Autodesk Fusion 360 part; units mm, degrees
note: some values were not read from the file. Chosen so that the rebuilt part matches the saved one: a direction. Set by a fixed rule: which sketch regions a step uses.
(part 2 of 8)
  arc A22 (27.5172, -41.7722) -> (27.7255, -40.9948) centre (13.5, -37.5997) ccw
  spline S11 degree 5 poles (27.7255, -40.9948) (27.7209, -40.9905) (27.7118, -40.9819) (27.698, -40.969) (27.6796, -40.952) (27.6566, -40.9308) (27.6336, -40.9097) (27.6104, -40.8888) (27.5872, -40.868) (27.564, -40.8473) (27.5406, -40.8268) (27.5173, -40.8064) (27.4938, -40.7861) (27.4703, -40.766) (27.4468, -40.746) (27.4232, -40.7262) (27.3995, -40.7065) (27.3758, -40.6869) (27.352, -40.6675) (27.3281, -40.6482) (27.3042, -40.6291) (27.2803, -40.6101) (27.2562, -40.5912) (27.2321, -40.5725) (27.208, -40.554) (27.1838, -40.5356) (27.1595, -40.5174) (27.1352, -40.4993) (27.1108, -40.4813) (27.0864, -40.4636) (27.0619, -40.4459) (27.0374, -40.4285) (27.0128, -40.4112) (26.9881, -40.394) (26.9634, -40.377) (26.9386, -40.3602) (26.9138, -40.3436) (26.8889, -40.3271) (26.8639, -40.3108) (26.8389, -40.2947) (26.8138, -40.2787) (26.7887, -40.2629) (26.7635, -40.2474) (26.7382, -40.232) (26.7129, -40.2167) (26.6876, -40.2017) (26.6621, -40.1869) (26.6367, -40.1722) (26.6111, -40.1577) (26.5855, -40.1435) (26.5599, -40.1294) (26.5341, -40.1156) (26.5083, -40.102) (26.4825, -40.0886) (26.4566, -40.0755) (26.4306, -40.0626) (26.4046, -40.0498) (26.3785, -40.0373) (26.3523, -40.025) (26.3261, -40.013) (26.2998, -40.0012) (26.2734, -39.9898) (26.247, -39.9788) (26.2204, -39.9682) (26.1937, -39.9578) (26.167, -39.9477) (26.1403, -39.9378) (26.1135, -39.9281) (26.0867, -39.9186) (26.0598, -39.9097) (26.0327, -39.9015) (26.0108, -39.8958) (25.9943, -39.8921) (25.9832, -39.8899) (25.9776, -39.8889) knots -1 -1 -1 -1 -1 -1 -0.98571429 -0.97142857 -0.95714286 -0.94285714 -0.92857143 -0.91428571 -0.9 -0.88571429 -0.87142857 -0.85714286 -0.84285714 -0.82857143 -0.81428571 -0.8 -0.78571429 -0.77142857 -0.75714286 -0.74285714 -0.72857143 -0.71428571 -0.7 -0.68571429 -0.67142857 -0.65714286 -0.64285714 -0.62857143 -0.61428571 -0.6 -0.58571429 -0.57142857 -0.55714286 -0.54285714 -0.52857143 -0.51428571 -0.5 -0.48571429 -0.47142857 -0.45714286 -0.44285714 -0.42857143 -0.41428571 -0.4 -0.38571429 -0.37142857 -0.35714286 -0.34285714 -0.32857143 -0.31428571 -0.3 -0.28571429 -0.27142857 -0.25714286 -0.24285714 -0.22857143 -0.21428571 -0.2 -0.18571429 -0.17142857 -0.15714286 -0.14285714 -0.12857143 -0.11428571 -0.1 -0.08571429 -0.07142857 -0.05714286 -0.04285714 -0.02857143 -0.01428571 0 0 0 0 0 0
  line L11 (25.9776, -39.8889) -> (25.5961, -39.8189)
  arc A23 (25.5156, -39.7033) -> (25.5961, -39.8189) centre (25.6141, -39.7205) ccw
  arc A24 (25.5156, -39.7033) -> (25.6507, -38.6777) centre (13.5, -37.5997) ccw
  arc A25 (25.7583, -38.5868) -> (25.6507, -38.6777) centre (25.7503, -38.6865) ccw
  line L12 (25.7583, -38.5868) -> (26.1449, -38.618)
  spline S12 degree 5 poles (26.1449, -38.618) (26.1506, -38.6184) (26.1618, -38.6192) (26.1788, -38.6199) (26.2014, -38.6201) (26.2297, -38.6192) (26.258, -38.6175) (26.2864, -38.6153) (26.3147, -38.6128) (26.3431, -38.6102) (26.3715, -38.6073) (26.3999, -38.6043) (26.4284, -38.6008) (26.4568, -38.5971) (26.4852, -38.5929) (26.5137, -38.5883) (26.5421, -38.5835) (26.5705, -38.5784) (26.599, -38.573) (26.6274, -38.5675) (26.6559, -38.5617) (26.6843, -38.5557) (26.7127, -38.5495) (26.7412, -38.5431) (26.7696, -38.5364) (26.798, -38.5294) (26.8264, -38.5223) (26.8549, -38.5149) (26.8833, -38.5073) (26.9117, -38.4996) (26.9401, -38.4916) (26.9684, -38.4835) (26.9968, -38.4751) (27.0252, -38.4666) (27.0535, -38.4579) (27.0819, -38.4489) (27.1102, -38.4398) (27.1385, -38.4305) (27.1669, -38.4211) (27.1952, -38.4114) (27.2234, -38.4016) (27.2517, -38.3916) (27.28, -38.3814) (27.3082, -38.3711) (27.3365, -38.3606) (27.3647, -38.3499) (27.3929, -38.339) (27.4211, -38.328) (27.4492, -38.3168) (27.4774, -38.3055) (27.5055, -38.294) (27.5337, -38.2823) (27.5618, -38.2705) (27.5898, -38.2585) (27.6179, -38.2464) (27.646, -38.2341) (27.674, -38.2216) (27.702, -38.209) (27.73, -38.1963) (27.7579, -38.1834) (27.7859, -38.1703) (27.8138, -38.1571) (27.8417, -38.1437) (27.8696, -38.1302) (27.8975, -38.1166) (27.9253, -38.1028) (27.9531, -38.0889) (27.9809, -38.0748) (28.0087, -38.0605) (28.0364, -38.0462) (28.0641, -38.0317) (28.0863, -38.0199) (28.1029, -38.0111) (28.1139, -38.0051) (28.1195, -38.0022) knots 0 0 0 0 0 0 0.01428571 0.02857143 0.04285714 0.05714286 0.07142857 0.08571429 0.1 0.11428571 0.12857143 0.14285714 0.15714286 0.17142857 0.18571429 0.2 0.21428571 0.22857143 0.24285714 0.25714286 0.27142857 0.28571429 0.3 0.31428571 0.32857143 0.34285714 0.35714286 0.37142857 0.38571429 0.4 0.41428571 0.42857143 0.44285714 0.45714286 0.47142857 0.48571429 0.5 0.51428571 0.52857143 0.54285714 0.55714286 0.57142857 0.58571429 0.6 0.61428571 0.62857143 0.64285714 0.65714286 0.67142857 0.68571429 0.7 0.71428571 0.72857143 0.74285714 0.75714286 0.77142857 0.78571429 0.8 0.81428571 0.82857143 0.84285714 0.85714286 0.87142857 0.88571429 0.9 0.91428571 0.92857143 0.94285714 0.95714286 0.97142857 0.98571429 1 1 1 1 1 1
  arc A26 (28.1195, -38.0022) -> (28.1195, -37.1973) centre (13.5, -37.5997) ccw
  spline S13 degree 5 poles (28.1195, -37.1973) (28.1139, -37.1943) (28.1029, -37.1884) (28.0863, -37.1795) (28.0641, -37.1678) (28.0364, -37.1533) (28.0087, -37.1389) (27.9809, -37.1247) (27.9531, -37.1106) (27.9253, -37.0966) (27.8975, -37.0828) (27.8696, -37.0692) (27.8417, -37.0557) (27.8138, -37.0423) (27.7859, -37.0291) (27.7579, -37.0161) (27.73, -37.0032) (27.702, -36.9904) (27.674, -36.9778) (27.646, -36.9653) (27.6179, -36.9531) (27.5898, -36.9409) (27.5618, -36.9289) (27.5337, -36.9171) (27.5055, -36.9054) (27.4774, -36.8939) (27.4492, -36.8826) (27.4211, -36.8714) (27.3929, -36.8604) (27.3647, -36.8495) (27.3365, -36.8389) (27.3082, -36.8283) (27.28, -36.818) (27.2517, -36.8078) (27.2234, -36.7978) (27.1952, -36.788) (27.1669, -36.7784) (27.1385, -36.7689) (27.1102, -36.7596) (27.0819, -36.7505) (27.0535, -36.7416) (27.0252, -36.7328) (26.9968, -36.7243) (26.9684, -36.716) (26.9401, -36.7078) (26.9117, -36.6999) (26.8833, -36.6921) (26.8549, -36.6845) (26.8264, -36.6772) (26.798, -36.67) (26.7696, -36.6631) (26.7412, -36.6564) (26.7127, -36.6499) (26.6843, -36.6437) (26.6559, -36.6377) (26.6274, -36.632) (26.599, -36.6264) (26.5705, -36.6211) (26.5421, -36.6159) (26.5137, -36.6111) (26.4852, -36.6066) (26.4568, -36.6024) (26.4284, -36.5986) (26.3999, -36.5952) (26.3715, -36.5921) (26.3431, -36.5893) (26.3147, -36.5866) (26.2864, -36.5841) (26.258, -36.5819) (26.2297, -36.5802) (26.2014, -36.5793) (26.1788, -36.5795) (26.1618, -36.5802) (26.1506, -36.581) (26.1449, -36.5815) knots -1 -1 -1 -1 -1 -1 -0.98571429 -0.97142857 -0.95714286 -0.94285714 -0.92857143 -0.91428571 -0.9 -0.88571429 -0.87142857 -0.85714286 -0.84285714 -0.82857143 -0.81428571 -0.8 -0.78571429 -0.77142857 -0.75714286 -0.74285714 -0.72857143 -0.71428571 -0.7 -0.68571429 -0.67142857 -0.65714286 -0.64285714 -0.62857143 -0.61428571 -0.6 -0.58571429 -0.57142857 -0.55714286 -0.54285714 -0.52857143 -0.51428571 -0.5 -0.48571429 -0.47142857 -0.45714286 -0.44285714 -0.42857143 -0.41428571 -0.4 -0.38571429 -0.37142857 -0.35714286 -0.34285714 -0.32857143 -0.31428571 -0.3 -0.28571429 -0.27142857 -0.25714286 -0.24285714 -0.22857143 -0.21428571 -0.2 -0.18571429 -0.17142857 -0.15714286 -0.14285714 -0.12857143 -0.11428571 -0.1 -0.08571429 -0.07142857 -0.05714286 -0.04285714 -0.02857143 -0.01428571 0 0 0 0 0 0
  line L13 (26.1449, -36.5815) -> (25.7583, -36.6126)
  arc A27 (25.6507, -36.5217) -> (25.7583, -36.6126) centre (25.7503, -36.5129) ccw
  arc A28 (25.6507, -36.5217) -> (25.5156, -35.4961) centre (13.5, -37.5997) ccw
  arc A29 (25.5961, -35.3805) -> (25.5156, -35.4961) centre (25.6141, -35.4789) ccw
  line L14 (25.5961, -35.3805) -> (25.9776, -35.3105)
  spline S14 degree 5 poles (25.9776, -35.3105) (25.9832, -35.3095) (25.9943, -35.3073) (26.0108, -35.3037) (26.0327, -35.298) (26.0598, -35.2898) (26.0867, -35.2808) (26.1135, -35.2713) (26.1403, -35.2616) (26.167, -35.2517) (26.1937, -35.2416) (26.2204, -35.2313) (26.247, -35.2206) (26.2734, -35.2096) (26.2998, -35.1982) (26.3261, -35.1865) (26.3523, -35.1744) (26.3785, -35.1621) (26.4046, -35.1496) (26.4306, -35.1369) (26.4566, -35.124) (26.4825, -35.1108) (26.5083, -35.0974) (26.5341, -35.0838) (26.5599, -35.07) (26.5855, -35.056) (26.6111, -35.0417) (26.6367, -35.0272) (26.6621, -35.0126) (26.6876, -34.9977) (26.7129, -34.9827) (26.7382, -34.9675) (26.7635, -34.9521) (26.7887, -34.9365) (26.8138, -34.9207) (26.8389, -34.9048) (26.8639, -34.8886) (26.8889, -34.8723) (26.9138, -34.8558) (26.9386, -34.8392) (26.9634, -34.8224) (26.9881, -34.8054) (27.0128, -34.7883) (27.0374, -34.771) (27.0619, -34.7535) (27.0864, -34.7359) (27.1108, -34.7181) (27.1352, -34.7002) (27.1595, -34.6821) (27.1838, -34.6638) (27.208, -34.6454) (27.2321, -34.6269) (27.2562, -34.6082) (27.2803, -34.5894) (27.3042, -34.5704) (27.3281, -34.5512) (27.352, -34.5319) (27.3758, -34.5125) (27.3995, -34.493) (27.4232, -34.4733) (27.4468, -34.4534) (27.4703, -34.4334) (27.4938, -34.4133) (27.5173, -34.393) (27.5406, -34.3726) (27.564, -34.3521) (27.5872, -34.3315) (27.6104, -34.3107) (27.6336, -34.2897) (27.6566, -34.2687) (27.6796, -34.2475) (27.698, -34.2304) (27.7118, -34.2176) (27.7209, -34.209) (27.7255, -34.2047) knots 0 0 0 0 0 0 0.01428571 0.02857143 0.04285714 0.05714286 0.07142857 0.08571429 0.1 0.11428571 0.12857143 0.14285714 0.15714286 0.17142857 0.18571429 0.2 0.21428571 0.22857143 0.24285714 0.25714286 0.27142857 0.28571429 0.3 0.31428571 0.32857143 0.34285714 0.35714286 0.37142857 0.38571429 0.4 0.41428571 0.42857143 0.44285714 0.45714286 0.47142857 0.48571429 0.5 0.51428571 0.52857143 0.54285714 0.55714286 0.57142857 0.58571429 0.6 0.61428571 0.62857143 0.64285714 0.65714286 0.67142857 0.68571429 0.7 0.71428571 0.72857143 0.74285714 0.75714286 0.77142857 0.78571429 0.8 0.81428571 0.82857143 0.84285714 0.85714286 0.87142857 0.88571429 0.9 0.91428571 0.92857143 0.94285714 0.95714286 0.97142857 0.98571429 1 1 1 1 1 1
  arc A30 (27.7255, -34.2047) -> (27.5172, -33.4272) centre (13.5, -37.5997) ccw
  spline S15 degree 5 poles (27.5172, -33.4272) (27.511, -33.4257) (27.4988, -33.4229) (27.4805, -33.4186) (27.4561, -33.413) (27.4255, -33.4062) (27.395, -33.3995) (27.3645, -33.3929) (27.334, -33.3865) (27.3036, -33.3802) (27.2731, -33.3741) (27.2427, -33.3681) (27.2122, -33.3623) (27.1818, -33.3566) (27.1514, -33.3511) (27.1211, -33.3457) (27.0907, -33.3405) (27.0604, -33.3354) (27.03, -33.3305) (26.9998, -33.3257) (26.9695, -33.3211) (26.9392, -33.3166) (26.909, -33.3123) (26.8788, -33.3082) (26.8486, -33.3042) (26.8185, -33.3004) (26.7883, -33.2967) (26.7582, -33.2932) (26.7281, -33.2898) (26.6981, -33.2867) (26.6681, -33.2836) (26.6381, -33.2808) (26.6081, -33.2781) (26.5782, -33.2756) (26.5483, -33.2733) (26.5184, -33.2711) (26.4886, -33.2691) (26.4588, -33.2673) (26.429, -33.2656) (26.3993, -33.2642) (26.3696, -33.2629) (26.34, -33.2618) (26.3103, -33.2609) (26.2808, -33.2602) (26.2512, -33.2597) (26.2218, -33.2593) (26.1923, -33.2592) (26.1629, -33.2592) (26.1336, -33.2595) (26.1043, -33.2599) (26.075, -33.2606) (26.0458, -33.2615) (26.0167, -33.2626) (25.9876, -33.2639) (25.9586, -33.2655) (25.9296, -33.2673) (25.9007, -33.2693) (25.8719, -33.2715) (25.8431, -33.2739) (25.8144, -33.2766) (25.7857, -33.2796) (25.7572, -33.2829) (25.7287, -33.2866) (25.7004, -33.2907) (25.6722, -33.295) (25.644, -33.2996) (25.6159, -33.3044) (25.5878, -33.3094) (25.5599, -33.3146) (25.5321, -33.3203) (25.5045, -33.3267) (25.4827, -33.3328) (25.4665, -33.3378) (25.4558, -33.3415) (25.4505, -33.3434) knots -1 -1 -1 -1 -1 -1 -0.98571429 -0.97142857 -0.95714286 -0.94285714 -0.92857143 -0.91428571 -0.9 -0.88571429 -0.87142857 -0.85714286 -0.84285714 -0.82857143 -0.81428571 -0.8 -0.78571429 -0.77142857 -0.75714286 -0.74285714 -0.72857143 -0.71428571 -0.7 -0.68571429 -0.67142857 -0.65714286 -0.64285714 -0.62857143 -0.61428571 -0.6 -0.58571429 -0.57142857 -0.55714286 -0.54285714 -0.52857143 -0.51428571 -0.5 -0.48571429 -0.47142857 -0.45714286 -0.44285714 -0.42857143 -0.41428571 -0.4 -0.38571429 -0.37142857 -0.35714286 -0.34285714 -0.32857143 -0.31428571 -0.3 -0.28571429 -0.27142857 -0.25714286 -0.24285714 -0.22857143 -0.21428571 -0.2 -0.18571429 -0.17142857 -0.15714286 -0.14285714 -0.12857143 -0.11428571 -0.1 -0.08571429 -0.07142857 -0.05714286 -0.04285714 -0.02857143 -0.01428571 0 0 0 0 0 0
  line L15 (25.4505, -33.3434) -> (25.0851, -33.4735)
  arc A31 (24.9576, -33.4137) -> (25.0851, -33.4735) centre (25.0516, -33.3793) ccw
  arc A32 (24.9576, -33.4137) -> (24.5618, -32.4579) centre (13.5, -37.5997) ccw
  arc A33 (24.6096, -32.3255) -> (24.5618, -32.4579) centre (24.6524, -32.4158) ccw
  line L16 (24.6096, -32.3255) -> (24.96, -32.1591)
  spline S16 degree 5 poles (24.96, -32.1591) (24.9651, -32.1567) (24.9752, -32.1517) (24.9903, -32.1439) (25.0099, -32.1327) (25.034, -32.1178) (25.0577, -32.1021) (25.0811, -32.086) (25.1045, -32.0697) (25.1277, -32.0532) (25.1509, -32.0366) (25.174, -32.0197) (25.1969, -32.0025) (25.2196, -31.985) (25.2421, -31.9672) (25.2645, -31.9491) (25.2867, -31.9306) (25.3087, -31.912) (25.3307, -31.8931) (25.3526, -31.8741) (25.3743, -31.8549) (25.3959, -31.8355) (25.4175, -31.8159) (25.4389, -31.7961) (25.4601, -31.7761) (25.4813, -31.7559) (25.5023, -31.7355) (25.5232, -31.7149) (25.5441, -31.6941) (25.5648, -31.6732) (25.5854, -31.6521) (25.6059, -31.6309) (25.6263, -31.6094) (25.6466, -31.5879) (25.6668, -31.5661) (25.6869, -31.5442) (25.7069, -31.5222) (25.7267, -31.5) (25.7465, -31.4776) (25.7662, -31.4551) (25.7858, -31.4324) (25.8053, -31.4096) (25.8247, -31.3867) (25.844, -31.3636) (25.8632, -31.3404) (25.8822, -31.317) (25.9012, -31.2935) (25.9202, -31.2699) (25.939, -31.2461) (25.9577, -31.2222) (25.9763, -31.1982) (25.9948, -31.174) (26.0132, -31.1498) (26.0316, -31.1253) (26.0498, -31.1008) (26.0679, -31.0761) (26.086, -31.0513) (26.1039, -31.0264) (26.1218, -31.0014) (26.1396, -30.9762) (26.1572, -30.9509) (26.1748, -30.9255) (26.1923, -30.9) (26.2097, -30.8744) (26.227, -30.8486) (26.2442, -30.8228) (26.2613, -30.7968) (26.2783, -30.7707) (26.2953, -30.7445) (26.3121, -30.7182) (26.3289, -30.6917) (26.3422, -30.6705) (26.3521, -30.6545) (26.3587, -30.6439) (26.362, -30.6385) knots 0 0 0 0 0 0 0.01428571 0.02857143 0.04285714 0.05714286 0.07142857 0.08571429 0.1 0.11428571 0.12857143 0.14285714 0.15714286 0.17142857 0.18571429 0.2 0.21428571 0.22857143 0.24285714 0.25714286 0.27142857 0.28571429 0.3 0.31428571 0.32857143 0.34285714 0.35714286 0.37142857 0.38571429 0.4 0.41428571 0.42857143 0.44285714 0.45714286 0.47142857 0.48571429 0.5 0.51428571 0.52857143 0.54285714 0.55714286 0.57142857 0.58571429 0.6 0.61428571 0.62857143 0.64285714 0.65714286 0.67142857 0.68571429 0.7 0.71428571 0.72857143 0.74285714 0.75714286 0.77142857 0.78571429 0.8 0.81428571 0.82857143 0.84285714 0.85714286 0.87142857 0.88571429 0.9 0.91428571 0.92857143 0.94285714 0.95714286 0.97142857 0.98571429 1 1 1 1 1 1
  arc A34 (26.362, -30.6385) -> (25.9596, -29.9415) centre (13.5, -37.5997) ccw
  spline S17 degree 5 poles (25.9596, -29.9415) (25.9533, -29.9416) (25.9408, -29.942) (25.922, -29.9427) (25.8969, -29.9436) (25.8657, -29.9449) (25.8344, -29.9463) (25.8033, -29.9479) (25.7722, -29.9496) (25.7411, -29.9514) (25.7101, -29.9534) (25.6792, -29.9555) (25.6483, -29.9577) (25.6174, -29.9601) (25.5866, -29.9626) (25.5559, -29.9653) (25.5252, -29.9681) (25.4946, -29.971) (25.4641, -29.9741) (25.4336, -29.9774) (25.4031, -29.9807) (25.3728, -29.9843) (25.3424, -29.9879) (25.3122, -29.9917) (25.282, -29.9957) (25.2519, -29.9998) (25.2218, -30.0041) (25.1918, -30.0085) (25.1619, -30.013) (25.1321, -30.0177) (25.1023, -30.0226) (25.0726, -30.0276) (25.043, -30.0327) (25.0134, -30.0381) (24.9839, -30.0435) (24.9545, -30.0492) (24.9252, -30.055) (24.8959, -30.0609) (24.8667, -30.067) (24.8376, -30.0733) (24.8086, -30.0798) (24.7797, -30.0864) (24.7509, -30.0932) (24.7221, -30.1001) (24.6935, -30.1073) (24.6649, -30.1146) (24.6364, -30.1221) (24.608, -30.1297) (24.5798, -30.1375) (24.5516, -30.1456) (24.5235, -30.1538) (24.4955, -30.1622) (24.4677, -30.1708) (24.4399, -30.1796) (24.4123, -30.1887) (24.3848, -30.1979) (24.3574, -30.2073) (24.3301, -30.2169) (24.3029, -30.2267) (24.2758, -30.2367) (24.249, -30.247) (24.2222, -30.2576) (24.1957, -30.2685) (24.1694, -30.2798) (24.1433, -30.2913) (24.1173, -30.3031) (24.0913, -30.315) (24.0655, -30.327) (24.0399, -30.3393) (24.0145, -30.352) (23.9895, -30.3653) (23.97, -30.3768) (23.9557, -30.3859) (23.9463, -30.3922) (23.9417, -30.3954) knots -1 -1 -1 -1 -1 -1 -0.98571429 -0.97142857 -0.95714286 -0.94285714 -0.92857143 -0.91428571 -0.9 -0.88571429 -0.87142857 -0.85714286 -0.84285714 -0.82857143 -0.81428571 -0.8 -0.78571429 -0.77142857 -0.75714286 -0.74285714 -0.72857143 -0.71428571 -0.7 -0.68571429 -0.67142857 -0.65714286 -0.64285714 -0.62857143 -0.61428571 -0.6 -0.58571429 -0.57142857 -0.55714286 -0.54285714 -0.52857143 -0.51428571 -0.5 -0.48571429 -0.47142857 -0.45714286 -0.44285714 -0.42857143 -0.41428571 -0.4 -0.38571429 -0.37142857 -0.35714286 -0.34285714 -0.32857143 -0.31428571 -0.3 -0.28571429 -0.27142857 -0.25714286 -0.24285714 -0.22857143 -0.21428571 -0.2 -0.18571429 -0.17142857 -0.15714286 -0.14285714 -0.12857143 -0.11428571 -0.1 -0.08571429 -0.07142857 -0.05714286 -0.04285714 -0.02857143 -0.01428571 0 0 0 0 0 0
  line L17 (23.9417, -30.3954) -> (23.6224, -30.6157)
  arc A35 (23.4838, -30.5908) -> (23.6224, -30.6157) centre (23.5656, -30.5334) ccw
  arc A36 (23.4838, -30.5908) -> (22.854, -29.7701) centre (13.5, -37.5997) ccw
  arc A37 (22.8659, -29.6298) -> (22.854, -29.7701) centre (22.9307, -29.706) ccw
  line L18 (22.8659, -29.6298) -> (23.1613, -29.3784)
  spline S18 degree 5 poles (23.1613, -29.3784) (23.1656, -29.3748) (23.1742, -29.3673) (23.1867, -29.3559) (23.2028, -29.34) (23.2221, -29.3193) (23.241, -29.2981) (23.2595, -29.2765) (23.2778, -29.2547) (23.296, -29.2327) (23.314, -29.2107) (23.332, -29.1884) (23.3496, -29.1659) (23.3671, -29.1431) (23.3842, -29.12) (23.4011, -29.0967) (23.4178, -29.0732) (23.4343, -29.0495) (23.4506, -29.0256) (23.4668, -29.0015) (23.4828, -28.9774) (23.4987, -28.953) (23.5144, -28.9285) (23.53, -28.9038) (23.5453, -28.879) (23.5605, -28.854) (23.5756, -28.8288) (23.5904, -28.8035) (23.6052, -28.7781) (23.6198, -28.7525) (23.6342, -28.7268) (23.6485, -28.701) (23.6627, -28.675) (23.6767, -28.6489) (23.6906, -28.6227) (23.7043, -28.5964) (23.7179, -28.5699) (23.7314, -28.5433) (23.7447, -28.5166) (23.7579, -28.4897) (23.771, -28.4628) (23.7839, -28.4357) (23.7967, -28.4086) (23.8093, -28.3813) (23.8219, -28.3539) (23.8343, -28.3264) (23.8465, -28.2987) (23.8587, -28.271) (23.8707, -28.2432) (23.8826, -28.2153) (23.8943, -28.1872) (23.906, -28.1591) (23.9175, -28.1309) (23.9289, -28.1025) (23.9401, -28.0741) (23.9513, -28.0456) (23.9623, -28.017) (23.9732, -27.9882) (23.9839, -27.9594) (23.9946, -27.9305) (24.0051, -27.9015) (24.0155, -27.8725) (24.0258, -27.8433) (24.036, -27.814) (24.046, -27.7847) (24.056, -27.7552) (24.0658, -27.7257) (24.0754, -27.6961) (24.085, -27.6664) (24.0945, -27.6366) (24.1038, -27.6068) (24.1112, -27.5828) (24.1167, -27.5648) (24.1203, -27.5528) (24.1221, -27.5468) knots 0 0 0 0 0 0 0.01428571 0.02857143 0.04285714 0.05714286 0.07142857 0.08571429 0.1 0.11428571 0.12857143 0.14285714 0.15714286 0.17142857 0.18571429 0.2 0.21428571 0.22857143 0.24285714 0.25714286 0.27142857 0.28571429 0.3 0.31428571 0.32857143 0.34285714 0.35714286 0.37142857 0.38571429 0.4 0.41428571 0.42857143 0.44285714 0.45714286 0.47142857 0.48571429 0.5 0.51428571 0.52857143 0.54285714 0.55714286 0.57142857 0.58571429 0.6 0.61428571 0.62857143 0.64285714 0.65714286 0.67142857 0.68571429 0.7 0.71428571 0.72857143 0.74285714 0.75714286 0.77142857 0.78571429 0.8 0.81428571 0.82857143 0.84285714 0.85714286 0.87142857 0.88571429 0.9 0.91428571 0.92857143 0.94285714 0.95714286 0.97142857 0.98571429 1 1 1 1 1 1
  arc A38 (24.1221, -27.5468) -> (23.5529, -26.9776) centre (13.5, -37.5997) ccw
  spline S19 degree 5 poles (23.5529, -26.9776) (23.5469, -26.9794) (23.5349, -26.9831) (23.5169, -26.9885) (23.493, -26.9959) (23.4631, -27.0052) (23.4333, -27.0147) (23.4036, -27.0243) (23.374, -27.034) (23.3445, -27.0438) (23.315, -27.0537) (23.2857, -27.0637) (23.2564, -27.0739) (23.2273, -27.0842) (23.1982, -27.0946) (23.1692, -27.1051) (23.1403, -27.1158) (23.1115, -27.1265) (23.0828, -27.1374) (23.0541, -27.1485) (23.0256, -27.1596) (22.9972, -27.1709) (22.9688, -27.1822) (22.9406, -27.1937) (22.9125, -27.2054) (22.8845, -27.2171) (22.8565, -27.229) (22.8287, -27.241) (22.801, -27.2532) (22.7734, -27.2655) (22.7459, -27.2779) (22.7185, -27.2904) (22.6912, -27.303) (22.664, -27.3158) (22.6369, -27.3288) (22.61, -27.3418) (22.5831, -27.355) (22.5564, -27.3683) (22.5298, -27.3818) (22.5033, -27.3954) (22.477, -27.4091) (22.4508, -27.423) (22.4247, -27.437) (22.3987, -27.4512) (22.3729, -27.4655) (22.3472, -27.4799) (22.3216, -27.4945) (22.2962, -27.5093) (22.2709, -27.5242) (22.2457, -27.5392) (22.2207, -27.5544) (22.1959, -27.5698) (22.1712, -27.5853) (22.1467, -27.601) (22.1224, -27.6169) (22.0982, -27.6329) (22.0741, -27.6491) (22.0503, -27.6654) (22.0265, -27.6819) (22.003, -27.6986) (21.9797, -27.7155) (21.9566, -27.7327) (21.9338, -27.7501) (21.9113, -27.7678) (21.8891, -27.7857) (21.867, -27.8037) (21.845, -27.8219) (21.8232, -27.8403) (21.8016, -27.8588) (21.7804, -27.8776) (21.7597, -27.897) (21.7439, -27.9131) (21.7324, -27.9256) (21.725, -27.9341) (21.7213, -27.9384) knots -1 -1 -1 -1 -1 -1 -0.98571429 -0.97142857 -0.95714286 -0.94285714 -0.92857143 -0.91428571 -0.9 -0.88571429 -0.87142857 -0.85714286 -0.84285714 -0.82857143 -0.81428571 -0.8 -0.78571429 -0.77142857 -0.75714286 -0.74285714 -0.72857143 -0.71428571 -0.7 -0.68571429 -0.67142857 -0.65714286 -0.64285714 -0.62857143 -0.61428571 -0.6 -0.58571429 -0.57142857 -0.55714286 -0.54285714 -0.52857143 -0.51428571 -0.5 -0.48571429 -0.47142857 -0.45714286 -0.44285714 -0.42857143 -0.41428571 -0.4 -0.38571429 -0.37142857 -0.35714286 -0.34285714 -0.32857143 -0.31428571 -0.3 -0.28571429 -0.27142857 -0.25714286 -0.24285714 -0.22857143 -0.21428571 -0.2 -0.18571429 -0.17142857 -0.15714286 -0.14285714 -0.12857143 -0.11428571 -0.1 -0.08571429 -0.07142857 -0.05714286 -0.04285714 -0.02857143 -0.01428571 0 0 0 0 0 0
  line L19 (21.7213, -27.9384) -> (21.4699, -28.2338)
  arc A39 (21.3296, -28.2457) -> (21.4699, -28.2338) centre (21.3938, -28.169) ccw
  arc A40 (21.3296, -28.2457) -> (20.5089, -27.6159) centre (13.5, -37.5997) ccw
  arc A41 (20.484, -27.4773) -> (20.5089, -27.6159) centre (20.5663, -27.5341) ccw
  line L20 (20.484, -27.4773) -> (20.7043, -27.158)
  spline S20 degree 5 poles (20.7043, -27.158) (20.7075, -27.1534) (20.7138, -27.144) (20.7229, -27.1297) (20.7344, -27.1102) (20.7477, -27.0852) (20.7604, -27.0598) (20.7727, -27.0342) (20.7848, -27.0084) (20.7967, -26.9825) (20.8084, -26.9564) (20.8199, -26.9303) (20.8312, -26.904) (20.8421, -26.8775) (20.8527, -26.8508) (20.863, -26.8239) (20.873, -26.7968) (20.8828, -26.7696) (20.8924, -26.7423) (20.9018, -26.7149) (20.911, -26.6874) (20.9201, -26.6598) (20.9289, -26.6321) (20.9375, -26.6042) (20.9459, -26.5762) (20.9542, -26.5481) (20.9622, -26.52) (20.97, -26.4917) (20.9777, -26.4633) (20.9851, -26.4348) (20.9924, -26.4062) (20.9996, -26.3776) (21.0065, -26.3488) (21.0133, -26.32) (21.0199, -26.2911) (21.0264, -26.2621) (21.0327, -26.233) (21.0388, -26.2038) (21.0447, -26.1745) (21.0505, -26.1452) (21.0562, -26.1158) (21.0617, -26.0863) (21.067, -26.0568) (21.0721, -26.0271) (21.0771, -25.9974) (21.082, -25.9676) (21.0867, -25.9378) (21.0913, -25.9079) (21.0957, -25.8779) (21.0999, -25.8478) (21.104, -25.8177) (21.108, -25.7875) (21.1118, -25.7573) (21.1155, -25.727) (21.119, -25.6966) (21.1224, -25.6661) (21.1256, -25.6356) (21.1287, -25.6051) (21.1316, -25.5745) (21.1344, -25.5438) (21.1371, -25.5131) (21.1396, -25.4823) (21.142, -25.4514) (21.1442, -25.4205) (21.1464, -25.3896) (21.1483, -25.3586) (21.1502, -25.3275) (21.1519, -25.2964) (21.1534, -25.2653) (21.1548, -25.2341) (21.1561, -25.2028) (21.157, -25.1777) (21.1577, -25.1589) (21.1581, -25.1464) (21.1583, -25.1401) knots 0 0 0 0 0 0 0.01428571 0.02857143 0.04285714 0.05714286 0.07142857 0.08571429 0.1 0.11428571 0.12857143 0.14285714 0.15714286 0.17142857 0.18571429 0.2 0.21428571 0.22857143 0.24285714 0.25714286 0.27142857 0.28571429 0.3 0.31428571 0.32857143 0.34285714 0.35714286 0.37142857 0.38571429 0.4 0.41428571 0.42857143 0.44285714 0.45714286 0.47142857 0.48571429 0.5 0.51428571 0.52857143 0.54285714 0.55714286 0.57142857 0.58571429 0.6 0.61428571 0.62857143 0.64285714 0.65714286 0.67142857 0.68571429 0.7 0.71428571 0.72857143 0.74285714 0.75714286 0.77142857 0.78571429 0.8 0.81428571 0.82857143 0.84285714 0.85714286 0.87142857 0.88571429 0.9 0.91428571 0.92857143 0.94285714 0.95714286 0.97142857 0.98571429 1 1 1 1 1 1
  arc A42 (21.1583, -25.1401) -> (20.4612, -24.7377) centre (13.5, -37.5997) ccw
  spline S21 degree 5 poles (20.4612, -24.7377) (20.4559, -24.741) (20.4452, -24.7476) (20.4292, -24.7575) (20.408, -24.7709) (20.3816, -24.7876) (20.3552, -24.8044) (20.329, -24.8214) (20.3029, -24.8384) (20.277, -24.8555) (20.2511, -24.8727) (20.2253, -24.89) (20.1997, -24.9074) (20.1742, -24.9249) (20.1488, -24.9425) (20.1235, -24.9602) (20.0983, -24.9779) (20.0733, -24.9958) (20.0484, -25.0137) (20.0236, -25.0318) (19.9989, -25.0499) (19.9744, -25.0682) (19.95, -25.0865) (19.9257, -25.1049) (19.9015, -25.1234) (19.8775, -25.142) (19.8536, -25.1608) (19.8298, -25.1796) (19.8062, -25.1985) (19.7827, -25.2175) (19.7593, -25.2366) (19.7361, -25.2558) (19.713, -25.275) (19.6901, -25.2944) (19.6673, -25.3139) (19.6446, -25.3335) (19.6221, -25.3532) (19.5998, -25.373) (19.5775, -25.3929) (19.5555, -25.4129) (19.5336, -25.4329) (19.5119, -25.4531) (19.4903, -25.4734) (19.4689, -25.4938) (19.4476, -25.5143) (19.4265, -25.5349) (19.4056, -25.5557) (19.3848, -25.5765) (19.3643, -25.5974) (19.3439, -25.6184) (19.3236, -25.6396) (19.3036, -25.6609) (19.2838, -25.6823) (19.2642, -25.7038) (19.2448, -25.7254) (19.2256, -25.7472) (19.2066, -25.769) (19.1877, -25.791) (19.1691, -25.813) (19.1507, -25.8352) (19.1325, -25.8576) (19.1147, -25.8801) (19.0972, -25.9029) (19.08, -25.9258) (19.0631, -25.9488) (19.0465, -25.972) (19.03, -25.9953) (19.0137, -26.0186) (18.9976, -26.0421) (18.9819, -26.0657) (18.967, -26.0898) (18.9559, -26.1095) (18.948, -26.1245) (18.943, -26.1347) (18.9406, -26.1398) knots -1 -1 -1 -1 -1 -1 -0.98571429 -0.97142857 -0.95714286 -0.94285714 -0.92857143 -0.91428571 -0.9 -0.88571429 -0.87142857 -0.85714286 -0.84285714 -0.82857143 -0.81428571 -0.8 -0.78571429 -0.77142857 -0.75714286 -0.74285714 -0.72857143 -0.71428571 -0.7 -0.68571429 -0.67142857 -0.65714286 -0.64285714 -0.62857143 -0.61428571 -0.6 -0.58571429 -0.57142857 -0.55714286 -0.54285714 -0.52857143 -0.51428571 -0.5 -0.48571429 -0.47142857 -0.45714286 -0.44285714 -0.42857143 -0.41428571 -0.4 -0.38571429 -0.37142857 -0.35714286 -0.34285714 -0.32857143 -0.31428571 -0.3 -0.28571429 -0.27142857 -0.25714286 -0.24285714 -0.22857143 -0.21428571 -0.2 -0.18571429 -0.17142857 -0.15714286 -0.14285714 -0.12857143 -0.11428571 -0.1 -0.08571429 -0.07142857 -0.05714286 -0.04285714 -0.02857143 -0.01428571 0 0 0 0 0 0
  line L21 (18.9406, -26.1398) -> (18.7743, -26.4902)
  arc A43 (18.6418, -26.538) -> (18.7743, -26.4902) centre (18.6839, -26.4473) ccw
  arc A44 (18.6418, -26.538) -> (17.6861, -26.1421) centre (13.5, -37.5997) ccw
  arc A45 (17.6262, -26.0146) -> (17.6861, -26.1421) centre (17.7204, -26.0482) ccw
  line L22 (17.6262, -26.0146) -> (17.7563, -25.6492)
  spline S22 degree 5 poles (17.7563, -25.6492) (17.7582, -25.6439) (17.7619, -25.6332) (17.767, -25.617) (17.773, -25.5952) (17.7794, -25.5676) (17.7851, -25.5398) (17.7903, -25.5119) (17.7953, -25.4838) (17.8001, -25.4557) (17.8047, -25.4276) (17.8091, -25.3993) (17.8131, -25.371) (17.8168, -25.3425) (17.8201, -25.314) (17.8231, -25.2854) (17.8258, -25.2566) (17.8282, -25.2278) (17.8304, -25.199) (17.8324, -25.1701) (17.8342, -25.1411) (17.8358, -25.1121) (17.8371, -25.083) (17.8383, -25.0539) (17.8391, -25.0247) (17.8398, -24.9954) (17.8403, -24.9661) (17.8405, -24.9368) (17.8405, -24.9074) (17.8404, -24.878) (17.8401, -24.8485) (17.8395, -24.8189) (17.8388, -24.7894) (17.8379, -24.7598) (17.8368, -24.7301) (17.8355, -24.7004) (17.8341, -24.6707) (17.8324, -24.6409) (17.8306, -24.6111) (17.8286, -24.5813) (17.8264, -24.5514) (17.8241, -24.5215) (17.8216, -24.4916) (17.8189, -24.4616) (17.8161, -24.4316) (17.8131, -24.4016) (17.8099, -24.3716) (17.8065, -24.3415) (17.803, -24.3114) (17.7993, -24.2813) (17.7955, -24.2511) (17.7915, -24.2209) (17.7874, -24.1907) (17.7831, -24.1605) (17.7786, -24.1302) (17.774, -24.1) (17.7692, -24.0697) (17.7643, -24.0394) (17.7592, -24.009) (17.754, -23.9787) (17.7486, -23.9483) (17.7431, -23.9179) (17.7374, -23.8875) (17.7316, -23.8571) (17.7256, -23.8266) (17.7195, -23.7962) (17.7132, -23.7657) (17.7068, -23.7352) (17.7002, -23.7047) (17.6935, -23.6742) (17.6867, -23.6437) (17.6811, -23.6192) (17.6768, -23.6009) (17.674, -23.5887) (17.6725, -23.5826) knots 0 0 0 0 0 0 0.01428571 0.02857143 0.04285714 0.05714286 0.07142857 0.08571429 0.1 0.11428571 0.12857143 0.14285714 0.15714286 0.17142857 0.18571429 0.2 0.21428571 0.22857143 0.24285714 0.25714286 0.27142857 0.28571429 0.3 0.31428571 0.32857143 0.34285714 0.35714286 0.37142857 0.38571429 0.4 0.41428571 0.42857143 0.44285714 0.45714286 0.47142857 0.48571429 0.5 0.51428571 0.52857143 0.54285714 0.55714286 0.57142857 0.58571429 0.6 0.61428571 0.62857143 0.64285714 0.65714286 0.67142857 0.68571429 0.7 0.71428571 0.72857143 0.74285714 0.75714286 0.77142857 0.78571429 0.8 0.81428571 0.82857143 0.84285714 0.85714286 0.87142857 0.88571429 0.9 0.91428571 0.92857143 0.94285714 0.95714286 0.97142857 0.98571429 1 1 1 1 1 1
  arc A46 (17.6725, -23.5826) -> (16.8951, -23.3742) centre (13.5, -37.5997) ccw
  spline S23 degree 5 poles (16.8951, -23.3742) (16.8908, -23.3788) (16.8822, -23.388) (16.8693, -23.4017) (16.8522, -23.4201) (16.8311, -23.4431) (16.81, -23.4662) (16.7891, -23.4893) (16.7683, -23.5125) (16.7476, -23.5358) (16.7271, -23.5591) (16.7067, -23.5824) (16.6864, -23.6059) (16.6663, -23.6294) (16.6463, -23.6529) (16.6265, -23.6765) (16.6068, -23.7002) (16.5872, -23.7239) (16.5678, -23.7477) (16.5485, -23.7716) (16.5294, -23.7955) (16.5104, -23.8195) (16.4915, -23.8435) (16.4728, -23.8676) (16.4543, -23.8917) (16.4359, -23.9159) (16.4176, -23.9402) (16.3996, -23.9645) (16.3816, -23.9889) (16.3638, -24.0133) (16.3462, -24.0378) (16.3287, -24.0623) (16.3114, -24.087) (16.2943, -24.1116) (16.2773, -24.1363) (16.2605, -24.1611) (16.2439, -24.186) (16.2274, -24.2109) (16.2111, -24.2358) (16.195, -24.2608) (16.179, -24.2859) (16.1632, -24.311) (16.1476, -24.3362) (16.1322, -24.3615) (16.117, -24.3868) (16.102, -24.4121) (16.0871, -24.4376) (16.0725, -24.4631) (16.058, -24.4886) (16.0438, -24.5142) (16.0297, -24.5399) (16.0159, -24.5656) (16.0023, -24.5914) (15.9889, -24.6172) (15.9758, -24.6431) (15.9628, -24.6691) (15.9501, -24.6952) (15.9376, -24.7213) (15.9253, -24.7474) (15.9132, -24.7736) (15.9015, -24.7999) (15.8901, -24.8263) (15.8791, -24.8528) (15.8684, -24.8793) (15.8581, -24.906) (15.848, -24.9327) (15.8381, -24.9594) (15.8284, -24.9862) (15.8189, -25.013) (15.8099, -25.0399) (15.8018, -25.067) (15.7961, -25.0889) (15.7924, -25.1055) (15.7902, -25.1166) (15.7892, -25.1221) knots -1 -1 -1 -1 -1 -1 -0.98571429 -0.97142857 -0.95714286 -0.94285714 -0.92857143 -0.91428571 -0.9 -0.88571429 -0.87142857 -0.85714286 -0.84285714 -0.82857143 -0.81428571 -0.8 -0.78571429 -0.77142857 -0.75714286 -0.74285714 -0.72857143 -0.71428571 -0.7 -0.68571429 -0.67142857 -0.65714286 -0.64285714 -0.62857143 -0.61428571 -0.6 -0.58571429 -0.57142857 -0.55714286 -0.54285714 -0.52857143 -0.51428571 -0.5 -0.48571429 -0.47142857 -0.45714286 -0.44285714 -0.42857143 -0.41428571 -0.4 -0.38571429 -0.37142857 -0.35714286 -0.34285714 -0.32857143 -0.31428571 -0.3 -0.28571429 -0.27142857 -0.25714286 -0.24285714 -0.22857143 -0.21428571 -0.2 -0.18571429 -0.17142857 -0.15714286 -0.14285714 -0.12857143 -0.11428571 -0.1 -0.08571429 -0.07142857 -0.05714286 -0.04285714 -0.02857143 -0.01428571 0 0 0 0 0 0
  line L23 (15.7892, -25.1221) -> (15.7192, -25.5036)
  arc A47 (15.6036, -25.5841) -> (15.7192, -25.5036) centre (15.6208, -25.4856) ccw
  arc A48 (15.6036, -25.5841) -> (14.578, -25.4491) centre (13.5, -37.5997) ccw
  arc A49 (14.4871, -25.3414) -> (14.578, -25.4491) centre (14.5868, -25.3495) ccw
  line L24 (14.4871, -25.3414) -> (14.5183, -24.9548)
  spline S24 degree 5 poles (14.5183, -24.9548) (14.5187, -24.9492) (14.5195, -24.9379) (14.5202, -24.9209) (14.5204, -24.8983) (14.5195, -24.87) (14.5178, -24.8417) (14.5156, -24.8133) (14.5131, -24.785) (14.5105, -24.7566) (14.5076, -24.7282) (14.5045, -24.6998) (14.5011, -24.6713) (14.4973, -24.6429) (14.4932, -24.6145) (14.4886, -24.5861) (14.4838, -24.5576) (14.4787, -24.5292) (14.4733, -24.5007) (14.4678, -24.4723) (14.462, -24.4439) (14.456, -24.4154) (14.4498, -24.387) (14.4433, -24.3586) (14.4366, -24.3301) (14.4297, -24.3017) (14.4226, -24.2733) (14.4152, -24.2449) (14.4076, -24.2165) (14.3999, -24.1881) (14.3919, -24.1597) (14.3838, -24.1313) (14.3754, -24.1029) (14.3669, -24.0745) (14.3581, -24.0462) (14.3492, -24.0178) (14.3401, -23.9895) (14.3308, -23.9612) (14.3214, -23.9329) (14.3117, -23.9046) (14.3019, -23.8763) (14.2919, -23.848) (14.2817, -23.8197) (14.2714, -23.7915) (14.2609, -23.7633) (14.2502, -23.735) (14.2393, -23.7068) (14.2283, -23.6786) (14.2171, -23.6505) (14.2058, -23.6223) (14.1943, -23.5942) (14.1826, -23.5661) (14.1708, -23.538) (14.1588, -23.5099) (14.1467, -23.4818) (14.1344, -23.4538) (14.1219, -23.4257) (14.1093, -23.3977) (14.0966, -23.3697) (14.0837, -23.3418) (14.0706, -23.3138) (14.0574, -23.2859) (14.044, -23.258) (14.0305, -23.2301) (14.0169, -23.2023) (14.0031, -23.1744) (13.9891, -23.1466) (13.9751, -23.1188) (13.9608, -23.0911) (13.9465, -23.0633) (13.9319, -23.0356) (13.9202, -23.0135) (13.9114, -22.9968) (13.9054, -22.9858) (13.9024, -22.9803) knots 0 0 0 0 0 0 0.01428571 0.02857143 0.04285714 0.05714286 0.07142857 0.08571429 0.1 0.11428571 0.12857143 0.14285714 0.15714286 0.17142857 0.18571429 0.2 0.21428571 0.22857143 0.24285714 0.25714286 0.27142857 0.28571429 0.3 0.31428571 0.32857143 0.34285714 0.35714286 0.37142857 0.38571429 0.4 0.41428571 0.42857143 0.44285714 0.45714286 0.47142857 0.48571429 0.5 0.51428571 0.52857143 0.54285714 0.55714286 0.57142857 0.58571429 0.6 0.61428571 0.62857143 0.64285714 0.65714286 0.67142857 0.68571429 0.7 0.71428571 0.72857143 0.74285714 0.75714286 0.77142857 0.78571429 0.8 0.81428571 0.82857143 0.84285714 0.85714286 0.87142857 0.88571429 0.9 0.91428571 0.92857143 0.94285714 0.95714286 0.97142857 0.98571429 1 1 1 1 1 1
  arc A50 (13.9024, -22.9803) -> (13.0976, -22.9803) centre (13.5, -37.5997) ccw
  spline S25 degree 5 poles (13.0976, -22.9803) (13.0946, -22.9858) (13.0886, -22.9968) (13.0798, -23.0135) (13.0681, -23.0356) (13.0535, -23.0633) (13.0392, -23.0911) (13.0249, -23.1188) (13.0109, -23.1466) (12.9969, -23.1744) (12.9831, -23.2023) (12.9695, -23.2301) (12.956, -23.258) (12.9426, -23.2859) (12.9294, -23.3138) (12.9163, -23.3418) (12.9034, -23.3697) (12.8907, -23.3977) (12.8781, -23.4257) (12.8656, -23.4538) (12.8533, -23.4818) (12.8412, -23.5099) (12.8292, -23.538) (12.8174, -23.5661) (12.8057, -23.5942) (12.7942, -23.6223) (12.7829, -23.6505) (12.7717, -23.6786) (12.7607, -23.7068) (12.7498, -23.735) (12.7391, -23.7633) (12.7286, -23.7915) (12.7183, -23.8197) (12.7081, -23.848) (12.6981, -23.8763) (12.6883, -23.9046) (12.6786, -23.9329) (12.6692, -23.9612) (12.6599, -23.9895) (12.6508, -24.0178) (12.6419, -24.0462) (12.6331, -24.0745) (12.6246, -24.1029) (12.6162, -24.1313) (12.6081, -24.1597) (12.6001, -24.1881) (12.5924, -24.2165) (12.5848, -24.2449) (12.5774, -24.2733) (12.5703, -24.3017) (12.5634, -24.3301) (12.5567, -24.3586) (12.5502, -24.387) (12.544, -24.4154) (12.538, -24.4439) (12.5322, -24.4723) (12.5267, -24.5007) (12.5213, -24.5292) (12.5162, -24.5576) (12.5114, -24.5861) (12.5068, -24.6145) (12.5027, -24.6429) (12.4989, -24.6713) (12.4955, -24.6998) (12.4924, -24.7282) (12.4895, -24.7566) (12.4869, -24.785) (12.4844, -24.8133) (12.4822, -24.8417) (12.4805, -24.87) (12.4796, -24.8983) (12.4798, -24.9209) (12.4805, -24.9379) (12.4813, -24.9492) (12.4817, -24.9548) knots -1 -1 -1 -1 -1 -1 -0.98571429 -0.97142857 -0.95714286 -0.94285714 -0.92857143 -0.91428571 -0.9 -0.88571429 -0.87142857 -0.85714286 -0.84285714 -0.82857143 -0.81428571 -0.8 -0.78571429 -0.77142857 -0.75714286 -0.74285714 -0.72857143 -0.71428571 -0.7 -0.68571429 -0.67142857 -0.65714286 -0.64285714 -0.62857143 -0.61428571 -0.6 -0.58571429 -0.57142857 -0.55714286 -0.54285714 -0.52857143 -0.51428571 -0.5 -0.48571429 -0.47142857 -0.45714286 -0.44285714 -0.42857143 -0.41428571 -0.4 -0.38571429 -0.37142857 -0.35714286 -0.34285714 -0.32857143 -0.31428571 -0.3 -0.28571429 -0.27142857 -0.25714286 -0.24285714 -0.22857143 -0.21428571 -0.2 -0.18571429 -0.17142857 -0.15714286 -0.14285714 -0.12857143 -0.11428571 -0.1 -0.08571429 -0.07142857 -0.05714286 -0.04285714 -0.02857143 -0.01428571 0 0 0 0 0 0
  line L25 (12.4817, -24.9548) -> (12.5129, -25.3414)
  arc A51 (12.422, -25.4491) -> (12.5129, -25.3414) centre (12.4132, -25.3495) ccw
  arc A52 (12.422, -25.4491) -> (11.3964, -25.5841) centre (13.5, -37.5997) ccw
  arc A53 (11.2808, -25.5036) -> (11.3964, -25.5841) centre (11.3792, -25.4856) ccw
  line L26 (11.2808, -25.5036) -> (11.2108, -25.1221)
  spline S26 degree 5 poles (11.2108, -25.1221) (11.2098, -25.1166) (11.2076, -25.1055) (11.2039, -25.0889) (11.1982, -25.067) (11.1901, -25.0399) (11.1811, -25.013) (11.1716, -24.9862) (11.1619, -24.9594) (11.152, -24.9327) (11.1419, -24.906) (11.1316, -24.8793) (11.1209, -24.8528) (11.1099, -24.8263) (11.0985, -24.7999) (11.0868, -24.7736) (11.0747, -24.7474) (11.0624, -24.7213) (11.0499, -24.6952) (11.0372, -24.6691) (11.0242, -24.6431) (11.0111, -24.6172) (10.9977, -24.5914) (10.9841, -24.5656) (10.9703, -24.5399) (10.9562, -24.5142) (10.942, -24.4886) (10.9275, -24.4631) (10.9129, -24.4376) (10.898, -24.4121) (10.883, -24.3868) (10.8678, -24.3615) (10.8524, -24.3362) (10.8368, -24.311) (10.821, -24.2859) (10.805, -24.2608) (10.7889, -24.2358) (10.7726, -24.2109) (10.7561, -24.186) (10.7395, -24.1611) (10.7227, -24.1363) (10.7057, -24.1116) (10.6886, -24.087) (10.6713, -24.0623) (10.6538, -24.0378) (10.6362, -24.0133) (10.6184, -23.9889) (10.6004, -23.9645) (10.5824, -23.9402) (10.5641, -23.9159) (10.5457, -23.8917) (10.5272, -23.8676) (10.5085, -23.8435) (10.4896, -23.8195) (10.4706, -23.7955) (10.4515, -23.7716) (10.4322, -23.7477) (10.4128, -23.7239) (10.3932, -23.7002) (10.3735, -23.6765) (10.3537, -23.6529) (10.3337, -23.6294) (10.3136, -23.6059) (10.2933, -23.5824) (10.2729, -23.5591) (10.2524, -23.5358) (10.2317, -23.5125) (10.2109, -23.4893) (10.19, -23.4662) (10.1689, -23.4431) (10.1478, -23.4201) (10.1307, -23.4017) (10.1178, -23.388) (10.1092, -23.3788) (10.1049, -23.3742) knots 0 0 0 0 0 0 0.01428571 0.02857143 0.04285714 0.05714286 0.07142857 0.08571429 0.1 0.11428571 0.12857143 0.14285714 0.15714286 0.17142857 0.18571429 0.2 0.21428571 0.22857143 0.24285714 0.25714286 0.27142857 0.28571429 0.3 0.31428571 0.32857143 0.34285714 0.35714286 0.37142857 0.38571429 0.4 0.41428571 0.42857143 0.44285714 0.45714286 0.47142857 0.48571429 0.5 0.51428571 0.52857143 0.54285714 0.55714286 0.57142857 0.58571429 0.6 0.61428571 0.62857143 0.64285714 0.65714286 0.67142857 0.68571429 0.7 0.71428571 0.72857143 0.74285714 0.75714286 0.77142857 0.78571429 0.8 0.81428571 0.82857143 0.84285714 0.85714286 0.87142857 0.88571429 0.9 0.91428571 0.92857143 0.94285714 0.95714286 0.97142857 0.98571429 1 1 1 1 1 1
  arc A54 (10.1049, -23.3742) -> (9.3275, -23.5826) centre (13.5, -37.5997) ccw
  spline S27 degree 5 poles (9.3275, -23.5826) (9.326, -23.5887) (9.3232, -23.6009) (9.3189, -23.6192) (9.3133, -23.6437) (9.3065, -23.6742) (9.2998, -23.7047) (9.2932, -23.7352) (9.2868, -23.7657) (9.2805, -23.7962) (9.2744, -23.8266) (9.2684, -23.8571) (9.2626, -23.8875) (9.2569, -23.9179) (9.2514, -23.9483) (9.246, -23.9787) (9.2408, -24.009) (9.2357, -24.0394) (9.2308, -24.0697) (9.226, -24.1) (9.2214, -24.1302) (9.2169, -24.1605) (9.2126, -24.1907) (9.2085, -24.2209) (9.2045, -24.2511) (9.2007, -24.2813) (9.197, -24.3114) (9.1935, -24.3415) (9.1901, -24.3716) (9.1869, -24.4016) (9.1839, -24.4316) (9.1811, -24.4616) (9.1784, -24.4916) (9.1759, -24.5215) (9.1736, -24.5514) (9.1714, -24.5813) (9.1694, -24.6111) (9.1676, -24.6409) (9.1659, -24.6707) (9.1645, -24.7004) (9.1632, -24.7301) (9.1621, -24.7598) (9.1612, -24.7894) (9.1605, -24.8189) (9.1599, -24.8485) (9.1596, -24.878) (9.1595, -24.9074) (9.1595, -24.9368) (9.1597, -24.9661) (9.1602, -24.9954) (9.1609, -25.0247) (9.1617, -25.0539) (9.1629, -25.083) (9.1642, -25.1121) (9.1658, -25.1411) (9.1676, -25.1701) (9.1696, -25.199) (9.1718, -25.2278) (9.1742, -25.2566) (9.1769, -25.2854) (9.1799, -25.314) (9.1832, -25.3425) (9.1869, -25.371) (9.1909, -25.3993) (9.1953, -25.4276) (9.1999, -25.4557) (9.2047, -25.4838) (9.2097, -25.5119) (9.2149, -25.5398) (9.2206, -25.5676) (9.227, -25.5952) (9.233, -25.617) (9.2381, -25.6332) (9.2418, -25.6439) (9.2437, -25.6492) knots -1 -1 -1 -1 -1 -1 -0.98571429 -0.97142857 -0.95714286 -0.94285714 -0.92857143 -0.91428571 -0.9 -0.88571429 -0.87142857 -0.85714286 -0.84285714 -0.82857143 -0.81428571 -0.8 -0.78571429 -0.77142857 -0.75714286 -0.74285714 -0.72857143 -0.71428571 -0.7 -0.68571429 -0.67142857 -0.65714286 -0.64285714 -0.62857143 -0.61428571 -0.6 -0.58571429 -0.57142857 -0.55714286 -0.54285714 -0.52857143 -0.51428571 -0.5 -0.48571429 -0.47142857 -0.45714286 -0.44285714 -0.42857143 -0.41428571 -0.4 -0.38571429 -0.37142857 -0.35714286 -0.34285714 -0.32857143 -0.31428571 -0.3 -0.28571429 -0.27142857 -0.25714286 -0.24285714 -0.22857143 -0.21428571 -0.2 -0.18571429 -0.17142857 -0.15714286 -0.14285714 -0.12857143 -0.11428571 -0.1 -0.08571429 -0.07142857 -0.05714286 -0.04285714 -0.02857143 -0.01428571 0 0 0 0 0 0
  line L27 (9.2437, -25.6492) -> (9.3738, -26.0146)
  arc A55 (9.3139, -26.1421) -> (9.3738, -26.0146) centre (9.2796, -26.0482) ccw
  arc A56 (9.3139, -26.1421) -> (8.3582, -26.538) centre (13.5, -37.5997) ccw
  arc A57 (8.2257, -26.4902) -> (8.3582, -26.538) centre (8.3161, -26.4473) ccw
  line L28 (8.2257, -26.4902) -> (8.0594, -26.1398)
  spline S28 degree 5 poles (8.0594, -26.1398) (8.057, -26.1347) (8.052, -26.1245) (8.0441, -26.1095) (8.033, -26.0898) (8.0181, -26.0657) (8.0024, -26.0421) (7.9863, -26.0186) (7.97, -25.9953) (7.9535, -25.972) (7.9369, -25.9488) (7.92, -25.9258) (7.9028, -25.9029) (7.8853, -25.8801) (7.8675, -25.8576) (7.8493, -25.8352) (7.8309, -25.813) (7.8123, -25.791) (7.7934, -25.769) (7.7744, -25.7472) (7.7552, -25.7254) (7.7358, -25.7038) (7.7162, -25.6823) (7.6964, -25.6609) (7.6764, -25.6396) (7.6561, -25.6184) (7.6357, -25.5974) (7.6152, -25.5765) (7.5944, -25.5557) (7.5735, -25.5349) (7.5524, -25.5143) (7.5311, -25.4938) (7.5097, -25.4734) (7.4881, -25.4531) (7.4664, -25.4329) (7.4445, -25.4129) (7.4225, -25.3929) (7.4002, -25.373) (7.3779, -25.3532) (7.3554, -25.3335) (7.3327, -25.3139) (7.3099, -25.2944) (7.287, -25.275) (7.2639, -25.2558) (7.2407, -25.2366) (7.2173, -25.2175) (7.1938, -25.1985) (7.1702, -25.1796) (7.1464, -25.1608) (7.1225, -25.142) (7.0985, -25.1234) (7.0743, -25.1049) (7.05, -25.0865) (7.0256, -25.0682) (7.0011, -25.0499) (6.9764, -25.0318) (6.9516, -25.0137) (6.9267, -24.9958) (6.9017, -24.9779) (6.8765, -24.9602) (6.8512, -24.9425) (6.8258, -24.9249) (6.8003, -24.9074) (6.7747, -24.89) (6.7489, -24.8727) (6.723, -24.8555) (6.6971, -24.8384) (6.671, -24.8214) (6.6448, -24.8044) (6.6184, -24.7876) (6.592, -24.7709) (6.5708, -24.7575) (6.5548, -24.7476) (6.5441, -24.741) (6.5388, -24.7377) knots 0 0 0 0 0 0 0.01428571 0.02857143 0.04285714 0.05714286 0.07142857 0.08571429 0.1 0.11428571 0.12857143 0.14285714 0.15714286 0.17142857 0.18571429 0.2 0.21428571 0.22857143 0.24285714 0.25714286 0.27142857 0.28571429 0.3 0.31428571 0.32857143 0.34285714 0.35714286 0.37142857 0.38571429 0.4 0.41428571 0.42857143 0.44285714 0.45714286 0.47142857 0.48571429 0.5 0.51428571 0.52857143 0.54285714 0.55714286 0.57142857 0.58571429 0.6 0.61428571 0.62857143 0.64285714 0.65714286 0.67142857 0.68571429 0.7 0.71428571 0.72857143 0.74285714 0.75714286 0.77142857 0.78571429 0.8 0.81428571 0.82857143 0.84285714 0.85714286 0.87142857 0.88571429 0.9 0.91428571 0.92857143 0.94285714 0.95714286 0.97142857 0.98571429 1 1 1 1 1 1
  arc A58 (6.5388, -24.7377) -> (5.8417, -25.1401) centre (13.5, -37.5997) ccw
  spline S29 degree 5 poles (5.8417, -25.1401) (5.8419, -25.1464) (5.8423, -25.1589) (5.843, -25.1777) (5.8439, -25.2028) (5.8452, -25.2341) (5.8466, -25.2653) (5.8481, -25.2964) (5.8498, -25.3275) (5.8517, -25.3586) (5.8536, -25.3896) (5.8558, -25.4205) (5.858, -25.4514) (5.8604, -25.4823) (5.8629, -25.5131) (5.8656, -25.5438) (5.8684, -25.5745) (5.8713, -25.6051) (5.8744, -25.6356) (5.8776, -25.6661) (5.881, -25.6966) (5.8845, -25.727) (5.8882, -25.7573) (5.892, -25.7875) (5.896, -25.8177) (5.9001, -25.8478) (5.9043, -25.8779) (5.9087, -25.9079) (5.9133, -25.9378) (5.918, -25.9676) (5.9229, -25.9974) (5.9279, -26.0271) (5.933, -26.0568) (5.9383, -26.0863) (5.9438, -26.1158) (5.9495, -26.1452) (5.9553, -26.1745) (5.9612, -26.2038) (5.9673, -26.233) (5.9736, -26.2621) (5.9801, -26.2911) (5.9867, -26.32) (5.9935, -26.3488) (6.0004, -26.3776) (6.0076, -26.4062) (6.0149, -26.4348) (6.0223, -26.4633) (6.03, -26.4917) (6.0378, -26.52) (6.0458, -26.5481) (6.0541, -26.5762) (6.0625, -26.6042) (6.0711, -26.6321) (6.0799, -26.6598) (6.089, -26.6874) (6.0982, -26.7149) (6.1076, -26.7423) (6.1172, -26.7696) (6.127, -26.7968) (6.137, -26.8239) (6.1473, -26.8508) (6.1579, -26.8775) (6.1688, -26.904) (6.1801, -26.9303) (6.1916, -26.9564) (6.2033, -26.9825) (6.2152, -27.0084) (6.2273, -27.0342) (6.2396, -27.0598) (6.2523, -27.0852) (6.2656, -27.1102) (6.2771, -27.1297) (6.2862, -27.144) (6.2925, -27.1534) (6.2957, -27.158) knots -1 -1 -1 -1 -1 -1 -0.98571429 -0.97142857 -0.95714286 -0.94285714 -0.92857143 -0.91428571 -0.9 -0.88571429 -0.87142857 -0.85714286 -0.84285714 -0.82857143 -0.81428571 -0.8 -0.78571429 -0.77142857 -0.75714286 -0.74285714 -0.72857143 -0.71428571 -0.7 -0.68571429 -0.67142857 -0.65714286 -0.64285714 -0.62857143 -0.61428571 -0.6 -0.58571429 -0.57142857 -0.55714286 -0.54285714 -0.52857143 -0.51428571 -0.5 -0.48571429 -0.47142857 -0.45714286 -0.44285714 -0.42857143 -0.41428571 -0.4 -0.38571429 -0.37142857 -0.35714286 -0.34285714 -0.32857143 -0.31428571 -0.3 -0.28571429 -0.27142857 -0.25714286 -0.24285714 -0.22857143 -0.21428571 -0.2 -0.18571429 -0.17142857 -0.15714286 -0.14285714 -0.12857143 -0.11428571 -0.1 -0.08571429 -0.07142857 -0.05714286 -0.04285714 -0.02857143 -0.01428571 0 0 0 0 0 0
  line L29 (6.2957, -27.158) -> (6.516, -27.4773)
  arc A59 (6.4911, -27.6159) -> (6.516, -27.4773) centre (6.4337, -27.5341) ccw
  arc A60 (6.4911, -27.6159) -> (5.6704, -28.2457) centre (13.5, -37.5997) ccw
  arc A61 (5.5301, -28.2338) -> (5.6704, -28.2457) centre (5.6062, -28.169) ccw
  line L30 (5.5301, -28.2338) -> (5.2787, -27.9384)
  spline S30 degree 5 poles (5.2787, -27.9384) (5.275, -27.9341) (5.2676, -27.9256) (5.2561, -27.9131) (5.2403, -27.897) (5.2196, -27.8776) (5.1984, -27.8588) (5.1768, -27.8403) (5.155, -27.8219) (5.133, -27.8037) (5.1109, -27.7857) (5.0887, -27.7678) (5.0662, -27.7501) (5.0434, -27.7327) (5.0203, -27.7155) (4.997, -27.6986) (4.9735, -27.6819) (4.9497, -27.6654) (4.9259, -27.6491) (4.9018, -27.6329) (4.8776, -27.6169) (4.8533, -27.601) (4.8288, -27.5853) (4.8041, -27.5698) (4.7793, -27.5544) (4.7543, -27.5392) (4.7291, -27.5242) (4.7038, -27.5093) (4.6784, -27.4945) (4.6528, -27.4799) (4.6271, -27.4655) (4.6013, -27.4512) (4.5753, -27.437) (4.5492, -27.423) (4.523, -27.4091) (4.4967, -27.3954) (4.4702, -27.3818) (4.4436, -27.3683) (4.4169, -27.355) (4.39, -27.3418) (4.3631, -27.3288) (4.336, -27.3158) (4.3088, -27.303) (4.2815, -27.2904) (4.2541, -27.2779) (4.2266, -27.2655) (4.199, -27.2532) (4.1713, -27.241) (4.1435, -27.229) (4.1155, -27.2171) (4.0875, -27.2054) (4.0594, -27.1937) (4.0312, -27.1822) (4.0028, -27.1709) (3.9744, -27.1596) (3.9459, -27.1485) (3.9172, -27.1374) (3.8885, -27.1265) (3.8597, -27.1158) (3.8308, -27.1051) (3.8018, -27.0946) (3.7727, -27.0842) (3.7436, -27.0739) (3.7143, -27.0637) (3.685, -27.0537) (3.6555, -27.0438) (3.626, -27.034) (3.5964, -27.0243) (3.5667, -27.0147) (3.5369, -27.0052) (3.507, -26.9959) (3.4831, -26.9885) (3.4651, -26.9831) (3.4531, -26.9794) (3.4471, -26.9776) knots 0 0 0 0 0 0 0.01428571 0.02857143 0.04285714 0.05714286 0.07142857 0.08571429 0.1 0.11428571 0.12857143 0.14285714 0.15714286 0.17142857 0.18571429 0.2 0.21428571 0.22857143 0.24285714 0.25714286 0.27142857 0.28571429 0.3 0.31428571 0.32857143 0.34285714 0.35714286 0.37142857 0.38571429 0.4 0.41428571 0.42857143 0.44285714 0.45714286 0.47142857 0.48571429 0.5 0.51428571 0.52857143 0.54285714 0.55714286 0.57142857 0.58571429 0.6 0.61428571 0.62857143 0.64285714 0.65714286 0.67142857 0.68571429 0.7 0.71428571 0.72857143 0.74285714 0.75714286 0.77142857 0.78571429 0.8 0.81428571 0.82857143 0.84285714 0.85714286 0.87142857 0.88571429 0.9 0.91428571 0.92857143 0.94285714 0.95714286 0.97142857 0.98571429 1 1 1 1 1 1
  arc A62 (3.4471, -26.9776) -> (2.8779, -27.5468) centre (13.5, -37.5997) ccw